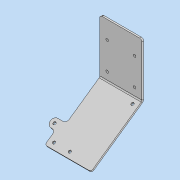
# Autodesk Inventor part: Fan_Holder
Saved by Autodesk Inventor 2020 (Build 240168000, 168)
## iProperties
Created: 2021-06-06
Part Number: Fan_Holder
Material: 一般
Document SubType Name: Sheet Metal
Designer: ken113
Density: 1 g/cm^3
Sheet Metal Rule: Default_mm
Appearance: 既定
Author: ken113
Autodesk Inventor part; units mm, degrees
ref_plane "YZ Plane" through (0, 0, 0) normal (1, 0, 0) x (0, 1, 0)
ref_plane "XZ Plane" through (0, 0, 0) normal (0, 1, 0) x (-1, 0, 0)
ref_plane "XY Plane" through (0, 0, 0) normal (0, 0, 1) x (1, 0, 0)
sketch "スケッチ1" plane through (0, 0, 0) normal (0, 0, 1) x (1, 0, 0)
  line L0 (20, 0) -> (-20, 0)
  line L1 (-20, 0) -> (-20, 50)
  line L2 (-20, 50) -> (20, 50)
  line L3 (20, 50) -> (20, 0)
  line L4 (20, 0) -> (-20, 50) construction
  line L5 (-20, 0) -> (20, 50) construction
  point P0 (0, 0)
  point P1 (0, 25)
  point P2 (0, 0)
  point P3 (0, 25)
  dimension "d0" = 40
  dimension "d1" = 50
  measures "d0" distance of L1.end L2.end
  measures "d1" distance of L0.end L1.end
extrude "プレート1" add sketch "スケッチ1" along normal blind 1.6
sketch "スケッチ2" plane through (20, -1.3106, 2.2823) normal (0, -0.819152, -0.5735764) x (1, 0, 0)
  line L0 (-40, 0) -> (0, 0)
  line L1 (0, 0) -> (0, 58.1342)
  line L2 (0, 58.1342) -> (-40, 58.1342)
  line L3 (-40, 58.1342) -> (-40, 0)
  constraints: 6 end point, 1 horizontal, 1 perpendicular, 1 vertical
edge flange "フランジ1" height 59.8 angle 55 thickness 1.6 bend radius 1.6 thickness toward (0, -0.819152, -0.5735764) relief straight relief width 1.6 relief depth 0.8 edges at (0, 0, 1.6) wall of the first edge with corners at (-20, -1.3106, 2.2823) (20, -1.3106, 2.2823) (20, -34.655, 49.903) (-20, -34.655, 49.903)
bend "曲げ1"
corner "コーナー1"
sketch "スケッチ3" plane through (0, 0, 0) normal (0, 0, -1) x (-1, 0, 0)
  line L0 (-20, 0) -> (20, 0) projected
  line L1 (20, 0) -> (20, 50) projected
  line L2 (20, 50) -> (-20, 50) projected
  line L3 (-20, 50) -> (-20, 0) projected
  line L4 (-20, 0) -> (20, 0) projected
  point P0 (0, 0)
  point P1 (-13, 7)
  point P2 (13, 7)
  point P3 (0, 7)
  point P4 (0, 0)
  point P5 (0, 0)
  point P6 (0, 7)
  point P7 (-13, 33)
  point P8 (13, 33)
  dimension "d62" = 7
  dimension "d85" = 26
  dimension "d86" = 13
  dimension "d90" = 26
  constraints: 4 vertical alignment, 3 horizontal alignment, 2 midpoint, 1 coincident
  measures "d62" distance from line of point (-13, 7) L0
  measures "d85" distance of point (13, 7) point (-13, 7)
  measures "d86" distance of point (0, 7) point (-13, 7)
  measures "d90" distance of point (13, 33) point (13, 7)
hole "穴1" at (13, 7, 0) at (-13, 7, 0) at (13, 33, 0) at (-13, 33, 0) direction (0, 0, 1) diameter 2.459 depth 8.8 tip angle 118 thread size "M3x0.5" class "6H" standard "ISO Metric profile"
sketch "スケッチ4" plane through (-20, -35.9657, 48.9853) normal (0, -0.819152, -0.5735764) x (1, 0, 0)
  line L0 (0, -58.1342) -> (40, -58.1342) projected
  line L1 (40, 0) -> (40, -58.1342) projected
  line L2 (0, 0) -> (40, 0) projected
  line L3 (0, -58.1342) -> (0, 0) projected
  point P0 (20, -60.7555)
  point P1 (35, -54.1342)
  dimension "d23" = 5
  dimension "d24" = 4
  measures "d23" distance from line of point (35, -54.134) L1
  measures "d24" distance from line of L0 point (35, -54.134)
hole "穴2" at (15, -4.9156, 4.6412) direction (0, 0.819152, 0.5735764) diameter 2.459 end through all thread size "M3x0.5" class "6H" standard "ISO Metric profile"
sketch "スケッチ5" plane through (-20, -35.9657, 48.9853) normal (0, -0.819152, -0.5735764) x (1, 0, 0)
  circle A0 centre (35, -54.1342) radius 1.2295 projected
  line L0 (0, 0) -> (0, -58.1342) projected
  line L1 (0, -12.1342) -> (-12, -12.1342)
  line L2 (-12, -12.1342) -> (-12, -20.1342)
  line L3 (-12, -20.1342) -> (0, -20.1342)
  line L4 (0, -20.1342) -> (0, -12.1342)
  point P0 (20, -60.7555)
  point P1 (-8, -16.1342)
  point P2 (0, -20.1342)
  dimension "d32" = 43
  dimension "d33" = 38
  dimension "d34" = 4
  dimension "d35" = 8
  dimension "d36" = 4
  constraints: 8 end point, 2 parallel, 1 horizontal, 1 perpendicular, 1 point on line
  measures "d32" horizontal distance of point (-8, -16.134) A0.centre
  measures "d33" vertical distance of point (-8, -16.134) A0.centre
  measures "d34" distance from line of point (-8, -16.134) L1
  measures "d35" distance of L1.end L2.end
  measures "d36" distance from line of point (-8, -16.134) L2
extrude "押し出し1" add sketch "スケッチ5" against normal up to surface (1.6 mm away) contours L0 L3 L2 L1
sketch "スケッチ6" plane through (-20, -35.9657, 48.9853) normal (0, -0.819152, -0.5735764) x (1, 0, 0)
  circle A0 centre (35, -54.1342) radius 1.2295 projected
  point P0 (20, -60.7555)
  point P1 (-8, -16.1342)
  dimension "d39" = 43
  dimension "d40" = 38
  measures "d39" horizontal distance of point (-8, -16.134) A0.centre
  measures "d40" vertical distance of point (-8, -16.134) A0.centre
hole "穴3" at (-28, -26.7115, 35.7689) direction (0, 0.819152, 0.5735764) diameter 2.459 depth 8.8 tip angle 118 thread size "M3x0.5" class "6H" standard "ISO Metric profile"
fillet "フィレット1" radius 4 2 edges at (-32, -23.7619, 32.9512) (-32, -28.3505, 39.5044)
fillet "フィレット2" radius 2 2 edges at (20, 50, 0.8) (-20, 50, 0.8)
sketch "スケッチ8" plane through (-20, -35.9657, 48.9853) normal (0, -0.819152, -0.5735764) x (1, 0, 0)
  line L0 (0, 0) -> (0, -12.1342) projected
  line L1 (0, 0) -> (-1, 0)
  line L2 (-1, 0) -> (-1, -12.1342)
  line L3 (-1, -12.1342) -> (0, -12.1342)
  line L4 (0, -12.1342) -> (0, 0)
  point P0 (20, -60.7555)
  point P1 (0, -12.1342)
  dimension "d63" = 1
  constraints: 8 end point, 2 parallel, 1 coincident, 1 horizontal, 1 perpendicular
  measures "d63" distance of L0.start L1.end
extrude "押し出し3" add sketch "スケッチ8" against normal up to surface (1.6 mm away)
sketch "スケッチ9" plane through (-20, -2.6213, 1.3646) normal (0, -0.819152, -0.5735764) x (1, 0, 0)
  line L0 (40, 58.1342) -> (-1, 58.1342) projected
  line L1 (-1, 58.1342) -> (-1, 46) projected
  point P0 (20, -2.6213)
  point P1 (1, 53.6342)
  point P2 (16, 53.6342)
  dimension "d66" = 4.5
  dimension "d67" = 15
  dimension "d68" = 2
  constraints: 1 horizontal alignment
  measures "d66" distance from line of point (1, 53.634) L0
  measures "d67" distance of point (1, 53.634) point (16, 53.634)
  measures "d68" distance from line of point (1, 53.634) L1
hole "穴4" at (-19, -33.3846, 45.2991) at (-4, -33.3846, 45.2991) direction (0, 0.819152, 0.5735764) diameter 2.459 end through all thread size "M3x0.5" class "6H" standard "ISO Metric profile"
sketch "スケッチ10" plane through (-20, -2.6213, 1.3646) normal (0, -0.819152, -0.5735764) x (1, 0, 0)
  line L0 (43, 58.1342) -> (-4, 58.1342)
  line L1 (-4, 58.1342) -> (-4, 50.1342)
  line L2 (-4, 50.1342) -> (43, 50.1342)
  line L3 (43, 50.1342) -> (43, 58.1342)
  line L4 (-1, 58.1342) -> (-1, 46) projected
  line L5 (40, 58.1342) -> (40, 0) projected
  line L6 (-1, 46) -> (-8, 46) projected
  line L7 (-4, 50.1342) -> (-1, 50.1342)
  line L8 (-1, 50.1342) -> (-1, 46)
  line L9 (-1, 46) -> (-4, 46)
  line L10 (-4, 46) -> (-4, 50.1342)
  point P0 (20, -2.6213)
  point P1 (-4, 46)
  dimension "d76" = 3
  dimension "d77" = 3
  dimension "d78" = 8
  constraints: 16 end point, 4 parallel, 2 horizontal, 2 perpendicular, 1 horizontal alignment
  measures "d76" distance between parallel lines of L1 L4
  measures "d77" distance between parallel lines of L5 L3
  measures "d78" distance of L0.end L1.end
extrude "押し出し4" add sketch "スケッチ10" against normal up to surface (1.6 mm away) contours L4 L2 L1 L0 | L4 L6 L10 L2
chamfer "面取り4" distance 2 angle 45 2 edges at (-20, -23.7619, 32.9512) (-24, -28.3505, 39.5044)
fillet "フィレット3" radius 2 6 edges at (-20, -22.6147, 31.3129) (-22, -23.7619, 32.9512) (-26, -28.3505, 39.5044) (-24, -29.4976, 41.1427) (-24, -35.3104, 49.4442) (20, -35.3104, 49.4442)
equation "\"d86\" = 0.5 * d85"
equation "\"d30\" = Thickness"
equation "\"d2\" = Thickness"
equation "\"d3\" = BendReliefWidth"
equation "\"d4\" = BendReliefDepth"
equation "\"d5\" = MinimumRemnant"
equation "\"d6\" = TransitionRadius"
equation "\"d9\" = BendRadius"
equation "\"d10\" = CornerReliefSize"
equation "\"d11\" = GapSize"
equation "\"d12\" = JacobiRadiusSize"
equation "\"BendRadius\" = Thickness"
equation "\"BendReliefWidth\" = Thickness"
equation "\"BendReliefDepth\" = 0.5 * Thickness"
equation "\"CornerReliefSize\" = 4 * Thickness"
equation "\"MinimumRemnant\" = 2 * Thickness"
equation "\"TransitionRadius\" = BendRadius"
equation "\"JacobiRadiusSize\" = BendRadius"
equation "\"GapSize\" = Thickness"
equation "\"Thickness\" = 1.6"
